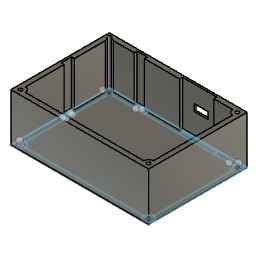
macronoxybase v2 v1 (Autodesk Fusion 360 design; units mm, degrees)
Autodesk Fusion 360 part; units mm, degrees
sketch "Sketch1" plane through (0, 0, 0) normal (0, 0, 1) x (1, 0, 0)
  line L0 (0, 0.9105) -> (0, 44.7087)
  line L1 (2.2913, 47) -> (17.5, 47)
  line L2 (17.5, 47) -> (15.35, 47)
  line L3 (0, 23.5) -> (0, 25.65)
  line L4 (0, 23.5) -> (0, 21.35)
  line L5 (-1.7, 23.5) -> (-1.7, 25.8)
  line L6 (-1.7, 23.5) -> (-1.7, 21.2)
  line L7 (70, 47) -> (74, 47) construction
  line L8 (0, 47) -> (-2.8284, 49.8284)
  line L9 (0, 47) -> (-4, 47) construction
  line L10 (-2.8284, 49.8284) -> (72.8284, 49.8284)
  line L11 (-2.8284, 49.8284) -> (-2.8284, -2.8284)
  line L12 (17.5, 47) -> (69, 47)
  line L13 (41.1957, 48.7475) -> (61.1957, 48.7475)
  line L14 (41.1957, 48.7475) -> (41.1957, 47)
  line L15 (61.1957, 48.7475) -> (61.1957, 47)
  line L16 (17.5, 48.7) -> (14.5, 48.7)
  line L17 (14.5, 48.7) -> (20.5, 48.7)
  line L18 (20.5, 48.7) -> (20.5, 47)
  line L19 (14.5, 48.7) -> (14.5, 47)
  line L20 (-1.7, 23.5) -> (-1.7, 26.5)
  line L21 (-1.7, 26.5) -> (-1.7, 23.5)
  line L22 (-1.7, 23.5) -> (-1.7, 20.5)
  line L23 (-1.7, 20.5) -> (-1.7, 26.5)
  line L24 (0, 26.5) -> (-1.7, 26.5)
  line L25 (-1.7, 20.5) -> (0, 20.5)
  line L26 (0, 47) -> (0, 48)
  line L27 (0, 48) -> (2.2913, 47)
  line L28 (0, 47) -> (-1, 47)
  line L29 (-1, 47) -> (0, 44.7087)
  arc A0 (0, 48) -> (-1, 47) centre (0, 47) ccw
  line L30 (-2.8284, 49.8284) -> (-2.8284, -7.8286)
  line L31 (-2.8284, 49.8284) -> (77.8286, 49.8284)
  line L32 (77.8286, 49.8284) -> (77.8286, -7.8286)
  line L33 (77.8286, -7.8286) -> (-2.8284, -7.8286)
  line L34 (0, -5) -> (75, -5)
  line L35 (75, -5) -> (75, 47)
  line L36 (75, 47) -> (69, 47)
  line L37 (0, 0.9105) -> (0, -5)
  circle A1 centre (75, 47) radius 2.8284
  circle A2 centre (75, 47) radius 1.05
  circle A3 centre (75, -5) radius 2.8286
  circle A4 centre (75, -5) radius 1.05
  circle A5 centre (0, -5) radius 2.8284
  circle A6 centre (0, -5) radius 1.05
  circle A7 centre (-0.7071, 47.7071) radius 1.05
  dimension "d2" = 47
  dimension "d3" = 17.5
  dimension "d5" = 2.15
  dimension "d23" = 2.15
  dimension "d25" = 1.7
  dimension "d26" = 2.3
  dimension "d27" = 2.3
  dimension "d33" = 45
  dimension "d34" = 4
  dimension "d59" = 6
  dimension "d60" = 3
  dimension "d61" = 3
  dimension "d63" = 2
  dimension "d70" = 20
  dimension "d72" = 2.5
  dimension "d73" = 2.5
  dimension "d126" = 57.657
  dimension "d127" = 80.657
  dimension "d128" = 2.1
  dimension "d129" = 2.1
  dimension "d130" = 2.1
  dimension "d131" = 2.1
  constraint perpendicular L0 L1
  constraint parallel L1 L2
  constraint parallel L0 L3
  constraint parallel L0 L4
  constraint horizontal L7
  constraint horizontal L9
  constraint coincident L12 L14.end
  constraint perpendicular L12 L14
  constraint coincident L12 L15.end
  constraint perpendicular L12 L15
  constraint coincident L12 L18.end
  constraint perpendicular L12 L18
  constraint coincident L1 L19.end
  constraint perpendicular L1 L19
  constraint coincident L0 L24.start
  constraint coincident L0 L25.end
  constraint perpendicular L0 L25
  constraint coincident L8.start L9.start
  constraint coincident L0 L3.start
  constraint perpendicular L9 L26
  constraint coincident L9 L28.end
  constraint perpendicular L9 L30
  constraint perpendicular L31 L32
  constraint perpendicular L30 L33
  constraint perpendicular L30 L34
  constraint perpendicular L7 L35
  constraint perpendicular L35 L36
  constraint perpendicular L34 L37
  constraint coincident L35.end L36.start
  constraint tangent L31 A1
  constraint coincident L34.end L35.start
  constraint tangent L32 A3
  constraint coincident L34.start L37.end
  constraint tangent L30 A5
  constraint concentric A5 A6
  constraint midpoint A0 A7.centre
  measures "d2" distance of origin L8.start
  measures "d3" distance of L8.start L1.end
  measures "d5" distance of L1.end L2.end
  measures "d23" distance of L3.start L3.end
  measures "d25" distance of L3.start L5.start
  measures "d26" distance of L5.start L5.end
  measures "d27" distance of L5.start L6.end
  measures "d33" angle of L8 L9
  measures "d34" distance of L8.start L8.end
  measures "d59" distance of L16.end L17.end
  measures "d60" distance of L5.start L20.end
  measures "d61" distance of L5.start L22.end
  measures "d63" diameter of A0
  measures "d70" horizontal distance of L13.start L13.end
  measures "d72" distance of L26.end L1.start
  measures "d73" distance of L28.end L0.end
  measures "d126" distance of L8.end L30.end
  measures "d127" distance of L8.end L31.end
  measures "d128" diameter of A2
  measures "d129" diameter of A4
  measures "d130" diameter of A6
  measures "d131" diameter of A7
sketch "Sketch2" plane through (0, 49.8284, 0) normal (0, 1, 0) x (-1, 0, 0)
  line L0 (-72.8284, 0) -> (2.8284, 0)
  line L1 (2.8284, 0) -> (2.8284, 28)
  line L2 (2.8284, 28) -> (-72.8284, 28)
  line L3 (-72.8284, 28) -> (-72.8284, 0)
  line L4 (-72.8284, 0) -> (-42.8284, 0)
  line L5 (-42.8284, 0) -> (-52.0284, 0)
  line L6 (-52.0284, 0) -> (-52.0284, 18)
  line L7 (-52.0284, 18) -> (-56.0284, 18)
  line L8 (-56.0284, 18) -> (-48.0284, 18)
  line L9 (-48.0284, 18) -> (-48.0284, 15)
  line L10 (-56.0284, 15) -> (-56.0284, 18)
  line L11 (-56.0284, 18) -> (-48, 18)
  line L12 (-48, 18) -> (-48, 14)
  line L13 (-48, 14) -> (-56.0284, 14)
  line L14 (-56.0284, 14) -> (-56.0284, 18)
  dimension "d49" = 30
  dimension "d50" = 9.2
  dimension "d51" = 18
  dimension "d52" = 4
  dimension "d53" = 8
  dimension "d54" = 3
  constraint coincident L0.start L3.end
  constraint perpendicular L3 L4
  constraint parallel L4 L5
  constraint perpendicular L4 L6
  constraint perpendicular L6 L7
  constraint horizontal L8
  constraint vertical L9
  constraint vertical L10
  constraint horizontal L11
  constraint vertical L12
  constraint horizontal L13
  constraint vertical L14
  measures "d49" distance of L0.start L4.end
  measures "d50" distance of L4.end L5.end
  measures "d51" distance of L5.end L6.end
  measures "d52" distance of L6.end L7.end
  measures "d53" distance of L7.end L8.end
  measures "d54" distance of L7.end L10.start
extrude "Extrude25" add sketch "Sketch1" along normal blind 28 contours L0 L5 L6 L8 L11 L20 L21 L22 L23 L24 L25 L29 L30 L37 A5 A7 | L34 L37 A5 A6 | L34 L37 A5 A6 | L33 L34 A3 A5 | L30 L33 A5 | L34 L35 A3 A4 | L34 L35 A3 A4 | L32 L35 A1 A3 | L32 L33 A3 | L1 L8 L10 L12 L13 L14 L15 L16 L17 L18 L19 L27 L31 L36 A1 A7 | L35 L36 A1 A2 | L35 L36 A1 A2 | L31 L32 A1
extrude "Extrude26" add sketch "Sketch1" along normal blind 2
extrude "Extrude27" cut sketch "Sketch2" against normal blind 6 contours L6 L7 L8 L10 L11 L13 L14 | L6 L8 L11 L12 L13
equation "d3 = ( 35 / 2 ) * 1 mm"
equation "d50 = ( 18.4 / 2 ) * 1 mm"
